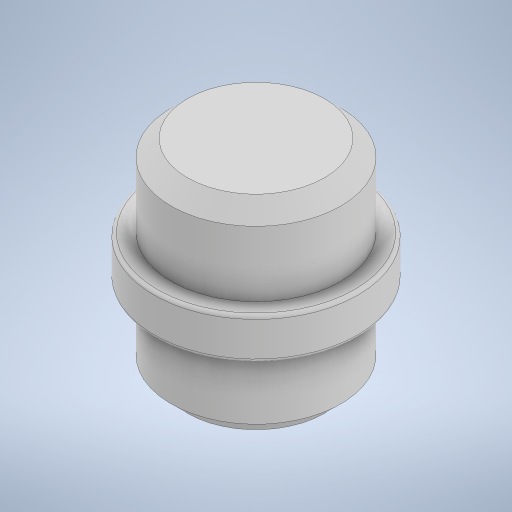
# Autodesk Inventor part: GuardStopper
Saved by Autodesk Inventor 2024 (Build 280153000, 153)
## iProperties
Created: 2025-01-06
Part Number: GuardStopper
Material: 常规
Document SubType Name: Modeling
Designer: nicx5
Density: 1 g/cm^3
Appearance: 默认
Author: nicx5
Autodesk Inventor part; units mm, degrees
ref_plane "YZ Plane" through (0, 0, 0) normal (1, 0, 0) x (0, 1, 0)
ref_plane "XZ Plane" through (0, 0, 0) normal (0, 1, 0) x (-1, 0, 0)
ref_plane "XY Plane" through (0, 0, 0) normal (0, 0, 1) x (1, 0, 0)
sketch "草图1" plane through (0, 0, 0) normal (0, 1, 0) x (-1, 0, 0)
  circle A0 centre (0, 0) radius 10.4
  dimension "d1" = 20.8
  constraints: 1 centre point
  measures "d1" diameter of A0
extrude "拉伸1" add sketch "草图1" along normal blind 10
sketch "草图2" plane through (0, 10, 0) normal (0, 1, 0) x (1, 0, 0)
  circle A0 centre (0, 0) radius 12.5
  dimension "d4" = 25
  constraints: 1 centre point, 1 coincident
  measures "d4" diameter of A0
extrude "拉伸2" add sketch "草图2" along normal blind 5
sketch "草图3" plane through (0, 15, 0) normal (0, 1, 0) x (1, 0, 0)
  circle A0 centre (0, 0) radius 10.4
  dimension "d7" = 20.8
  constraints: 1 centre point, 1 coincident
  measures "d7" diameter of A0
extrude "拉伸3" add sketch "草图3" along normal blind 10
chamfer "倒角1" distance 2 angle 45 2 edges at (10.4, 0, 0) (-10.4, 25, 0)
fillet "圆角1" radius 0.4 2 edges at (-12.5, 10, 0) (-12.5, 15, 0)
